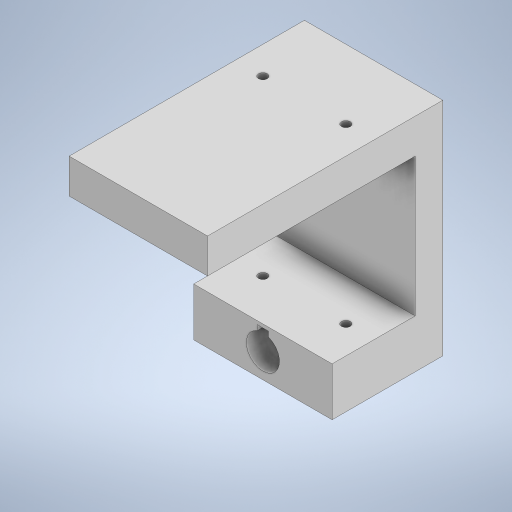
# Autodesk Inventor part: EndEffectorMotorAdapter
Saved by Autodesk Inventor 2024 (Build 280153000, 153)
## iProperties
Created: 2024-02-13
Part Number: EndEffectorMotorAdapter
Material: Generic
Document SubType Name: Modeling
Designer: yusuf
Density: 1 g/cm^3
Appearance: Default
Author: yusuf
Autodesk Inventor part; units mm, degrees
ref_plane "YZ Plane" through (0, 0, 0) normal (1, 0, 0) x (0, 1, 0)
ref_plane "XZ Plane" through (0, 0, 0) normal (0, 1, 0) x (-1, 0, 0)
ref_plane "XY Plane" through (0, 0, 0) normal (0, 0, 1) x (1, 0, 0)
sketch "Sketch1" plane through (0, 0, 0) normal (0, 0, 1) x (1, 0, 0)
  line L0 (0, 0) -> (100, 0)
  line L1 (100, 0) -> (100, 35)
  line L2 (100, 35) -> (0, 35)
  line L3 (0, 35) -> (0, 0)
  dimension "d0" = 100
  dimension "d1" = 35
  constraints: 8 end point, 2 parallel, 1 horizontal, 1 perpendicular
  measures "d0" distance of L1.end L2.end
  measures "d1" distance of L0.end L1.end
extrude "Extrusion1" add sketch "Sketch1" along normal blind 80
sketch "Sketch2" plane through (0, 0, 80) normal (0, 0, 1) x (1, 0, 0)
  circle A0 centre (50, 17.5) radius 12
  line L0 (100, 35) -> (0, 35) projected
  line L1 (0, 35) -> (0, 0) projected
  line L2 (50, 29.5) -> (50, 32.5)
  line L3 (50, 32.5) -> (54, 32.5)
  line L4 (54, 32.5) -> (54, 28.8137)
  line L5 (50, 32.5) -> (46, 32.5)
  line L6 (46, 32.5) -> (46, 28.8137)
  point P0 (0, 17.5)
  dimension "d4" = 17.5
  dimension "d5" = 50
  dimension "d6" = 24
  dimension "d7" = 3
  dimension "d8" = 4
  dimension "d9" = 4
  dimension "d10" = 2.5
  constraints: 10 end point, 3 point on circle, 2 horizontal, 2 perpendicular, 1 centre point, 1 midpoint, 1 vertical
  measures "d4" distance from line of L0 A0.centre
  measures "d5" distance of A0.centre point (0, 17.5)
  measures "d6" diameter of A0
  measures "d7" distance of L2.start L2.end
  measures "d8" distance of L2.end L3.end
  measures "d9" distance of L2.end L5.end
  measures "d10" distance between parallel lines of L5 L0
extrude "Extrusion2" cut sketch "Sketch2" against normal blind 40
sketch "Sketch3" plane through (0, 35, 0) normal (0, 1, 0) x (1, 0, 0)
  line L0 (100, 0) -> (100, -80) projected
  line L1 (0, 0) -> (100, 0)
  line L2 (100, 0) -> (100, -20)
  line L3 (100, -20) -> (0, -20)
  line L4 (0, -20) -> (0, 0)
  dimension "d13" = 20
  constraints: 8 end point, 2 parallel, 1 horizontal, 1 perpendicular, 1 point on line
  measures "d13" distance of L0.start L2.end
extrude "Extrusion3" add sketch "Sketch3" along normal blind 125
sketch "Sketch4" plane through (0, 35, 20) normal (0, 0, 1) x (1, 0, 0)
  line L0 (0, 0) -> (0, 125) projected
  line L1 (0, 125) -> (100, 125)
  line L2 (100, 125) -> (100, 100)
  line L3 (100, 100) -> (0, 100)
  line L4 (0, 100) -> (0, 125)
  point P0 (0, -35)
  point P1 (0, 100)
  dimension "d16" = 25
  dimension "d17" = 100
  constraints: 8 end point, 2 parallel, 1 horizontal, 1 perpendicular
  measures "d16" distance of L1.end L2.end
  measures "d17" distance between parallel lines of L0 L2
extrude "Extrusion4" add sketch "Sketch4" along normal blind 150
sketch "Sketch5" plane through (0, 35, 80) normal (0, 1, 0) x (1, 0, 0)
  circle A0 centre (20, 30) radius 3.175
  line L0 (100, 0) -> (0, 0) projected
  line L1 (0, 60) -> (0, 0) projected
  circle A1 centre (80, 30) radius 3.175
  line L2 (100, 60) -> (100, 0) projected
  point P0 (0, 80)
  dimension "d20" = 6.35
  dimension "d21" = 30
  dimension "d22" = 20
  dimension "d23" = 6.35
  dimension "d24" = 20
  dimension "d25" = 30
  constraints: 2 centre point
  measures "d20" diameter of A0
  measures "d21" distance from line of L0 A0.centre
  measures "d22" distance from line of L1 A0.centre
  measures "d23" diameter of A1
  measures "d24" distance from line of L2 A1.centre
  measures "d25" distance from line of L0 A1.centre
extrude "Extrusion5" cut sketch "Sketch5" along normal mid plane 300
equation "\"d23\" = d20"
equation "\"d24\" = d22"
equation "\"d25\" = d21"
body "Solid1"
